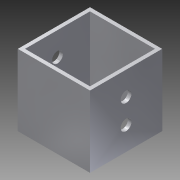
# Autodesk Inventor part: Square pipe
Saved by Autodesk Inventor 2015 (Build 190159000, 159)
## iProperties
Created: 2015-06-23
Part Number: Square pipe
Material: アルミニウム 6061
Document SubType Name: Modeling
Designer: kenta
Density: 2.7 g/cm^3
Appearance: アルミニウム - フラット - Version 1.1
Author: kenta
Autodesk Inventor part; units mm, degrees
ref_plane "YZ Plane" through (0, 0, 0) normal (1, 0, 0) x (0, 1, 0)
ref_plane "XZ Plane" through (0, 0, 0) normal (0, 1, 0) x (-1, 0, 0)
ref_plane "XY Plane" through (0, 0, 0) normal (0, 0, 1) x (1, 0, 0)
sketch "スケッチ1" plane through (0, 0, 0) normal (0, 0, 1) x (1, 0, 0)
  line L0 (-18, 18) -> (18, 18)
  line L1 (18, 18) -> (18, -18)
  line L2 (18, -18) -> (-18, -18)
  line L3 (-18, -18) -> (-18, 18)
  line L4 (-18, 18) -> (18, -18) construction
  line L5 (18, 18) -> (-18, -18) construction
  line L6 (-20, 20) -> (20, 20)
  line L7 (20, 20) -> (20, -20)
  line L8 (20, -20) -> (-20, -20)
  line L9 (-20, -20) -> (-20, 20)
  line L10 (-20, 20) -> (20, -20) construction
  line L11 (20, 20) -> (-20, -20) construction
  point P0 (0, 0)
  dimension "d0" = 36
  dimension "d1" = 36
  dimension "d2" = 40
  dimension "d3" = 40
  constraints: 24 end point, 4 midpoint, 4 parallel, 2 horizontal, 2 perpendicular
  measures "d0" distance of L1.end L2.end
  measures "d1" distance of L0.end L1.end
  measures "d2" distance of L7.end L8.end
  measures "d3" distance of L6.end L7.end
extrude "押し出し1" add sketch "スケッチ1" along normal blind 39.5
sketch "スケッチ2" plane through (20, -20, 0) normal (1, 0, 0) x (0, 0, -1)
  line L0 (0, 40) -> (-39.5, 40) projected
  line L1 (0, 40) -> (0, 0) projected
  line L2 (-39.5, 0) -> (-39.5, 40) projected
  point P0 (0, 20)
  point P1 (-13, 20)
  point P2 (-26.5, 20)
  dimension "d13" = 13.5
  dimension "d14" = 20
  dimension "d15" = 13
  dimension "d16" = 13
  dimension "d17" = 20
  constraints: 1 horizontal alignment
  measures "d13" distance of point (-13, 20) point (-26.5, 20)
  measures "d14" distance from line of point (-13, 20) L0
  measures "d15" distance from line of point (-13, 20) L1
  measures "d16" distance from line of point (-26.5, 20) L2
  measures "d17" distance from line of point (-26.5, 20) L0
hole "穴1" at (20, 0, 13) at (20, 0, 26.5) direction (-1, 0, 0) diameter 6 end through all
